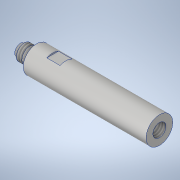
# Autodesk Inventor part: kicker_mitte
Saved by Autodesk Inventor 2020 (Build 240168000, 168)
## iProperties
Part Number: kicker_mitte
Material: Aluminum 6061
Document SubType Name: Modeling
Designer: rYan
Mass: 21.4287 g
Surface Area: 15.1763 cm^2
Volume: 2.72978 cm^3
Density: 2.7 g/cm^3
Appearance: Aluminum - Flat
Author: rYan
Autodesk Inventor part; units mm, degrees
ref_plane "YZ Plane" through (0, 0, 0) normal (1, 0, 0) x (0, 1, 0)
ref_plane "XZ Plane" through (0, 0, 0) normal (0, 1, 0) x (-1, 0, 0)
ref_plane "XY Plane" through (0, 0, 0) normal (0, 0, 1) x (1, 0, 0)
sketch "Skizze1" plane through (0, 0, 0) normal (0, 0, 1) x (1, 0, 0)
  line L0 (0, 0) -> (52, 0)
  line L1 (0, 0) -> (0, 3)
  line L2 (0, 3) -> (6, 3)
  line L3 (6, 3) -> (6, 5)
  line L4 (6, 5) -> (52, 5)
  line L5 (52, 5) -> (52, 0)
  dimension "d1" = 6
  dimension "d2" = 10
  dimension "d3" = 6
  dimension "d17" = 46
  constraints: 12 end point, 2 perpendicular, 2 vertical, 1 coincident, 1 horizontal, 1 parallel
  measures "d1" diameter of L2 L0
  measures "d2" diameter of L4 L0
  measures "d3" distance of L1.end L2.end
  measures "d17" distance of L3.end L4.end
revolve "Umdrehung1" add sketch "Skizze1" angle 360 about axis through (0, 0, 0) along (1, 0, 0)
sketch "Skizze2" plane through (52, 0, 0) normal (1, 0, 0) x (0, 0, -1)
  point P0 (0, 0)
  point P1 (0, 0)
  constraints: 1 coincident
hole "Bohrung1" at (52, 0, 0) direction (-1, 0, 0) diameter 4.917 depth 13 tip angle 118 thread size "M6x1" class "6H" standard "ISO Metric profile"
sketch "Sketch3" plane through (6, 0, 0) normal (-1, 0, 0) x (0, 0, 1)
  circle A0 centre (0, 0) radius 3 projected
  circle A1 centre (0, 0) radius 2.2
  dimension "d21" = 4.4
  constraints: 1 centre point, 1 coincident
  measures "d21" diameter of A1
extrude "Extrusion1" cut sketch "Sketch3" along normal blind 1.1
chamfer "Chamfer6" distance 1.4 distance2 0.8 1 edges at (4.9, -3, 0) measured on face at (4.4, -3, 0)
chamfer "Chamfer7" distance 1.4 distance2 0.8 1 edges at (0, -3, 0) measured on face at (0.5, -3, 0)
fillet "Fillet3" radius 0.6 3 edges at (4.9, -2.2001, 0) (4.9, 0, -2.2) (6, 0, -2.2)
thread "Thread3" size "M6x1" class "6g" standard "ANSI Metric M Profile" full length
sketch "Sketch4" plane through (0, 0, 0) normal (0, 1, 0) x (-1, 0, 0)
  line L0 (-6, 5) -> (-6, -5) projected
  line L1 (-52, 5) -> (-52, -5) projected
  line L2 (-6, 5) -> (-52, 5) projected
  line L3 (-17, 5) -> (-12, 5)
  line L4 (-12, 5) -> (-12, 4.5)
  line L5 (-12, 4.5) -> (-17, 4.5)
  line L6 (-17, 4.5) -> (-17, 5)
  line L7 (-6, -5) -> (-52, -5) projected
  line L8 (-17, -5) -> (-12, -5)
  line L9 (-12, -5) -> (-12, -4.5)
  line L10 (-12, -4.5) -> (-17, -4.5)
  line L11 (-17, -4.5) -> (-17, -5)
  point P0 (0, 0)
  point P1 (-12, -5)
  point P2 (-12, 5)
  dimension "d46" = 5
  dimension "d47" = 0.5
  dimension "d48" = 5
  dimension "d49" = 0.5
  dimension "d50" = 35
  dimension "d51" = 35
  constraints: 16 end point, 4 parallel, 2 horizontal, 2 perpendicular, 2 point on line
  measures "d46" distance of L4.end L5.end
  measures "d47" distance of L3.end L4.end
  measures "d48" distance of L10.end L9.end
  measures "d49" distance of L9.end L8.end
  measures "d50" distance from line of L1 L8.start
  measures "d51" distance from line of L1 L3.start
extrude "Extrusion2" cut sketch "Sketch4" against normal through all both and the other way through all contours L4 L5 L6 L2 | L7 L11 L10 L9
